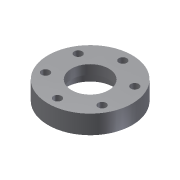
# Autodesk Inventor part: nylon clamp
Saved by Autodesk Inventor 2011 (Build 150239000, 239)
## iProperties
Created: 2011-05-26
Part Number: nylon clamp
Document SubType Name: Modeling
Designer: ijs09
Density: 1 g/cm^3
Author: ijs09
Autodesk Inventor part; units mm, degrees
ref_plane "YZ Plane" through (0, 0, 0) normal (1, 0, 0) x (0, 1, 0)
ref_plane "XZ Plane" through (0, 0, 0) normal (0, 1, 0) x (-1, 0, 0)
ref_plane "XY Plane" through (0, 0, 0) normal (0, 0, 1) x (1, 0, 0)
sketch "Sketch1" plane through (0, 0, 0) normal (0, 0, 1) x (1, 0, 0)
  circle A0 centre (0, 0) radius 22.5
  dimension "d0" = 45
  constraints: 1 centre point, 1 coincident
  measures "d0" diameter of A0
extrude "Extrusion1" add sketch "Sketch1" along normal blind 10
sketch "Sketch4" plane through (0, 0, 10) normal (0, 0, 1) x (1, 0, 0)
  circle A0 centre (0, 0) radius 22.5 projected
  circle A1 centre (0, 0) radius 17.5
  point P0 (0, 17.5)
  point P1 (-15.1554, 8.75)
  point P2 (-15.1554, -8.75)
  point P3 (0, -17.5)
  point P4 (15.1554, -8.75)
  point P5 (15.1554, 8.75)
  dimension "d18" = 35
  dimension "d21" = 360
  constraints: 1 coincident, 1 vertical alignment, 9 other
hole "Hole3" at (0, 17.5, 10) at (-15.1554, 8.75, 10) at (-15.1554, -8.75, 10) at (0, -17.5, 10) at (15.1554, -8.75, 10) at (15.1554, 8.75, 10) direction (0, 0, -1) diameter 4.3 end through all
sketch "Sketch5" plane through (0, 0, 0) normal (0, 0, -1) x (-1, 0, 0)
  circle A0 centre (0, 0) radius 22.5 projected
hole "Hole4" at (0, 0, 0) direction (0, 0, 1) diameter 25.5 depth 5
sketch "Sketch6" plane through (0, 0, 5) normal (0, 0, -1) x (-1, 0, 0)
  circle A0 centre (0, 0) radius 12.75 projected
  constraints: 1 coincident
hole "Hole5" at (0, 0, 5) at (0, 0, 5) direction (0, 0, 1) diameter 20 end through all
body "Solid1"
